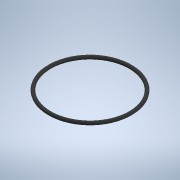
# Autodesk Inventor part: 2-038
Saved by Autodesk Inventor 2021 (Build 250183000, 183)
## iProperties
Created: 2021-10-18
Part Number: 2-038
Material: Rubber
Document SubType Name: Modeling
Designer: Alex Clay
Density: 0.93 g/cm^3
Appearance: Rubber - Black
Mass: 0.310286 g
Surface Area: 7.50598 cm^2
Volume: 0.333641 cm^3
Author: ALEX CLAY
Comments: PARKER SIZE 2-030
Autodesk Inventor part; units mm, degrees
ref_plane "YZ Plane" through (0, 0, 0) normal (1, 0, 0) x (0, 1, 0)
ref_plane "XZ Plane" through (0, 0, 0) normal (0, 1, 0) x (-1, 0, 0)
ref_plane "XY Plane" through (0, 0, 0) normal (0, 0, 1) x (1, 0, 0)
sketch "Sketch1" plane through (0, 0, 0) normal (0, 0, 1) x (1, 0, 0)
  circle A0 centre (21.3868, 0) radius 0.889
  line L0 (20.4978, 5.952) -> (20.4978, -5.6627) construction
  line L1 (-4.4552, 0) -> (26.731, 0) projected
  line L2 (0, -7.9856) -> (0, 8.2749) projected
  point P0 (0, 0)
  dimension "d0" = 1.778
  dimension "d1" = 20.4978
  constraints: 2 end point, 1 centre point, 1 point on line, 1 tangent, 1 vertical
  measures "d0" diameter of A0
  measures "d1" distance from line of L0 point (0, 0)
revolve "Revolution1" add sketch "Sketch1" angle 360 about axis through (0, -10, 0) along (0, 1, 0)
body "Solid1"
